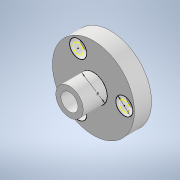
# Autodesk Inventor part: Bearing_Mount
Saved by Autodesk Inventor 2022 (Build 260153070, 153G)
## iProperties
Created: 2022-03-05
Part Number: Bearing_Mount
Material: Generic
Document SubType Name: Modeling
Designer: a laptop
Density: 1 g/cm^3
Appearance: Default
Author: a laptop
Autodesk Inventor part; units mm, degrees
ref_plane "YZ Plane" through (0, 0, 0) normal (1, 0, 0) x (0, 1, 0)
ref_plane "XZ Plane" through (0, 0, 0) normal (0, 1, 0) x (-1, 0, 0)
ref_plane "XY Plane" through (0, 0, 0) normal (0, 0, 1) x (1, 0, 0)
sketch "Sketch1" plane through (0, 0, 0) normal (0, 0, 1) x (1, 0, 0)
  circle A0 centre (0, 0) radius 12
  circle A1 centre (0, 0) radius 9 construction
  circle A2 centre (9, 0) radius 1.5
  circle A3 centre (-4.5, -7.7942) radius 1.5
  circle A4 centre (-4.5, 7.7942) radius 1.5
  line L0 (9, 0) -> (-4.5, -7.7942) construction
  line L1 (-4.5, 7.7942) -> (-4.5, -7.7942) construction
  line L2 (9, 0) -> (-4.5, 7.7942) construction
  circle A5 centre (0, 0) radius 2.5
  dimension "d0" = 24
  dimension "d1" = 18
  dimension "d2" = 3
  dimension "d3" = 5
  constraints: 6 centre point, 6 end point, 3 point on circle, 2 coincident, 2 equal length, 2 equal radius, 1 concentric, 1 vertical
  measures "d0" diameter of A0
  measures "d1" diameter of A1
  measures "d2" diameter of A4
  measures "d3" diameter of A5
extrude "Extrusion1" add sketch "Sketch1" along normal blind 5
sketch "Sketch2" plane through (0, 0, 5) normal (0, 0, 1) x (1, 0, 0)
  circle A0 centre (9, 0) radius 2.5
  circle A1 centre (-4.5, 7.7942) radius 2.5
  circle A2 centre (-4.5, -7.7942) radius 2.5
  circle A3 centre (9, 0) radius 1.5 projected
  circle A4 centre (-4.5, -7.7942) radius 1.5 projected
  circle A5 centre (-4.5, 7.7942) radius 1.5 projected
  circle A6 centre (0, 0) radius 4
  circle A7 centre (0, 0) radius 2.5 projected
  circle A8 centre (0, 0) radius 6.5
  dimension "d6" = 5
  dimension "d7" = 8
  dimension "d12" = 13
  constraints: 5 centre point, 3 concentric, 2 coincident, 2 equal radius
  measures "d6" diameter of A0
  measures "d7" diameter of A6
  measures "d12" diameter of A8
extrude "Extrusion2" cut sketch "Sketch2" against normal blind 3 contours A0 | A2 | A1 | A5
extrude "Extrusion3" add sketch "Sketch2" along normal blind 9 contours A6
sketch "Sketch3" plane through (0, 0, 0) normal (0, 0, -1) x (-1, 0, 0)
  circle A0 centre (0, 0) radius 12 projected
  circle A1 centre (0, 0) radius 5.5
  dimension "d13" = 11
  constraints: 1 centre point, 1 coincident
  measures "d13" diameter of A1
extrude "Extrusion4" cut sketch "Sketch3" against normal blind 3 contours A1
body "Solid1"
